frame_hanger (Autodesk Fusion 360 design; units mm, degrees)
Autodesk Fusion 360 part; units mm, degrees
sketch "Sketch1" plane through (0, 0, 0) normal (0, 1, 0) x (1, 0, 0)
  line L0 (0, 0) -> (27, 0)
  line L1 (27, 0) -> (53, -9.4632)
  line L2 (53, -9.4632) -> (53, 0)
  line L3 (0, -2) -> (26.6473, -2)
  line L4 (26.6473, -2) -> (52.316, -11.3426)
  line L5 (53, -9.4632) -> (52.316, -11.3426)
  line L6 (0, -2) -> (0, 0)
  line L7 (53, 0) -> (27, 0)
  line L8 (53, -9.4632) -> (56.4443, 0)
  line L9 (56.4443, 0) -> (53, 0)
  dimension "d1" = 27
  dimension "d3" = 160
  dimension "d4" = 26
  dimension "d5" = 2
  constraint coincident L0.start L6.end
  constraint horizontal L0
  constraint perpendicular L0 L2
  constraint perpendicular L0 L6
  constraint perpendicular L2 L7
  constraint perpendicular L1 L8
  constraint collinear L7 L9
  measures "d1" distance of L0.start L0.end
  measures "d3" angle of L0 L1
  measures "d4" horizontal distance of L0.end L1.end
extrude "Extrude1" add sketch "Sketch1" along normal blind 20
sketch "Sketch2" plane through (2.4744, 0, -6.7982) normal (-0.34202, 0, 0.939693) x (0, -1, 0)
  line L0 (0, 25.7244) -> (0, 53.0403)
  line L1 (0, 53.0403) -> (-20, 53.0403)
  line L2 (-20, 53.0403) -> (-20, 25.7244)
  line L3 (-20, 25.7244) -> (0, 25.7244)
  line L4 (-17.5, 25.7244) -> (-11.4522, 49.1091)
  line L5 (-8.5478, 49.1091) -> (-2.5, 25.7244)
  line L6 (-10, 25.7244) -> (-10, 53.0403)
  arc A0 (-8.5478, 49.1091) -> (-11.4522, 49.1091) centre (-10, 48.7335) ccw
  point P0 (-10, 54.7244)
  dimension "d8" = 7.5
  dimension "d9" = 7.5
  dimension "d10" = 29
  dimension "d11" = 1.5
  constraint coincident L3 L4.start
  constraint coincident L3 L5.end
  constraint midpoint L3 L6.start
  constraint midpoint L1 L6.end
  constraint coincident P0 L6
  constraint coincident P0 L4
  constraint coincident P0 L5
  constraint tangent L4 A0
  constraint tangent L5 A0
  measures "d8" distance of L4.start L6.start
  measures "d9" distance of L5.end L6.start
  measures "d10" distance of P0 L6.start
  measures "d11" radius of A0
extrude "Extrude2" cut sketch "Sketch2" against normal blind 15 contours L3 L5 L6 A0 | L3 L4 L6 A0
sketch "Sketch3" plane through (0, 20, 0) normal (0, 1, 0) x (-1, 0, 0)
  line L0 (-52.316, 11.3426) -> (-56.4443, 0)
  line L1 (-56.4443, 0) -> (0, 0)
  line L2 (0, 0) -> (0, 2)
  line L3 (0, 2) -> (-26.6473, 2)
  line L4 (-26.6473, 2) -> (-52.316, 11.3426)
  line L5 (-56.4443, 5) -> (-17.3231, 5)
  line L6 (-17.3231, 5) -> (-17.3231, 14.1022)
  line L7 (-17.3231, 14.1022) -> (-56.4443, 14.1022)
  line L8 (-56.4443, 14.1022) -> (-56.4443, 5)
  line L9 (-56.4443, 0) -> (-56.4443, 5)
  dimension "d14" = 5
  constraint horizontal L5
  constraint vertical L6
  constraint horizontal L7
  constraint vertical L8
  constraint coincident L0.end L1.start
  constraint coincident L5 L8.end
  constraint perpendicular L5 L9
  constraint coincident L5.start L8.end
  measures "d14" distance of L1 L5
extrude "Extrude3" cut sketch "Sketch3" against normal blind 86 contours L0 L4 L5 | L0 L4 L5 L6 L7 L8
equation "d9 = d8"
